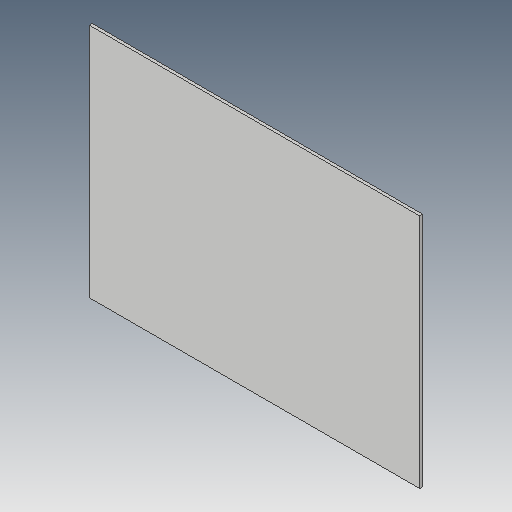
# Autodesk Inventor part: 防水p4
Saved by Autodesk Inventor 2020.3 (Build 243373000, 373)
## iProperties
Part Number: 防水p4
Material: 一般
Document SubType Name: Modeling
Designer: highs
Density: 1 g/cm^3
Appearance: 既定
Author: highs
Autodesk Inventor part; units mm, degrees
ref_plane "YZ Plane" through (0, 0, 0) normal (1, 0, 0) x (0, 1, 0)
ref_plane "XZ Plane" through (0, 0, 0) normal (0, 1, 0) x (-1, 0, 0)
ref_plane "XY Plane" through (0, 0, 0) normal (0, 0, 1) x (1, 0, 0)
sketch "スケッチ1" plane through (0, 0, 0) normal (0, 0, 1) x (1, 0, 0)
  line L0 (0, 0) -> (448, 0)
  line L1 (448, 0) -> (448, 320)
  line L2 (448, 320) -> (0, 320)
  line L3 (0, 320) -> (0, 0)
  dimension "d0" = 448
  dimension "d1" = 320
  constraints: 8 end point, 2 parallel, 1 horizontal, 1 perpendicular
  measures "d0" distance of L1.end L2.end
  measures "d1" distance of L2.end L0.start
extrude "押し出し1" add sketch "スケッチ1" along normal blind 4
